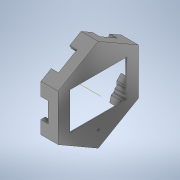
# Autodesk Inventor part: Hexagone
Saved by Autodesk Inventor 2020 (Build 240168000, 168)
## iProperties
Created: 2020-04-08
Part Number: Hexagone
Material: Silicon Nitride
Document SubType Name: Modeling
Designer: Samuele
Density: 3.18 g/cm^3
Appearance: Chrome - Polished Black
Author: Samuele
## iProperties of the stored document _3DPrint.ipt
Created: 2020-04-30
Part Number: _3DPrint
Material: Generic
Document SubType Name: Modeling
Designer: Samuele
Density: 1 g/cm^3
Appearance: Default
Author: Samuele
Autodesk Inventor part; units mm, degrees
ref_plane "YZ Plane" through (0, 0, 0) normal (1, 0, 0) x (0, 1, 0)
ref_plane "XZ Plane" through (0, 0, 0) normal (0, 1, 0) x (-1, 0, 0)
ref_plane "XY Plane" through (0, 0, 0) normal (0, 0, 1) x (1, 0, 0)
sketch "Sketch6" plane through (0, 0, 0) normal (0, 1, 0) x (-1, 0, 0)
  line L0 (4.5, -5.6) -> (60.5, -5.6)
  line L1 (60.5, -5.6) -> (60.5, -91.4)
  line L2 (4.5, -91.4) -> (4.5, -5.6)
  line L3 (65.1201, -97) -> (0, -97)
  line L4 (0, -97) -> (0, 0)
  line L5 (0, 0) -> (65.1201, 0)
  line L6 (65.1201, 0) -> (65.1201, -97)
  line L7 (60.5, -91.4) -> (4.5, -91.4)
  line L8 (102.5, -48.5) -> (-37.5, -48.5)
  line L9 (32.5, -118.5) -> (32.5, 21.5)
  circle A0 centre (32.5, -48.5) radius 70
  line L10 (102.5, -48.5) -> (67.5, -109.1218)
  line L11 (67.5, -109.1218) -> (-2.5, -109.1218)
  line L12 (-2.5, -109.1218) -> (-37.5, -48.5)
  line L13 (-37.5, -48.5) -> (-2.5, 12.1218)
  line L14 (-2.5, 12.1218) -> (67.5, 12.1218)
  line L15 (67.5, 12.1218) -> (102.5, -48.5)
  line L16 (32.5, 12.1218) -> (85, -18.1891)
  line L17 (85, -18.1891) -> (85, -78.8109)
  line L18 (85, -78.8109) -> (32.5, -109.1218)
  line L19 (32.5, -109.1218) -> (-20, -78.8109)
  line L20 (-20, -78.8109) -> (-20, -18.1891)
  line L21 (-20, -18.1891) -> (32.5, 12.1218)
  line L22 (32.5, 12.1218) -> (47.5, 12.1218)
  line L23 (47.5, 12.1218) -> (47.5, 5.6218)
  line L24 (47.5, 5.6218) -> (17.5, 5.6218)
  line L25 (17.5, 5.6218) -> (17.5, 12.1218)
  line L26 (47.5, 5.6218) -> (56.6924, 5.6218) construction
  line L27 (17.5, 8.8718) -> (19.5, 8.8718)
  line L28 (47.5, 8.8718) -> (45.5, 8.8718)
  line L29 (45.5, 8.8718) -> (45.5, 10.1218)
  line L30 (45.5, 10.1218) -> (19.5, 10.1218)
  line L31 (19.5, 10.1218) -> (19.5, 7.6218)
  line L32 (19.5, 7.6218) -> (45.5, 7.6218)
  line L33 (45.5, 7.6218) -> (45.5, 10.1218)
  line L34 (67.5, 12.1218) -> (32.5, -48.5)
  line L35 (32.5, -48.5) -> (67.5, -109.1218)
  line L36 (47.5, 5.6218) -> (56.6924, 5.6218)
  line L37 (17.5, 5.6218) -> (11, 5.6218)
  line L38 (17.5, 12.1218) -> (11, 5.6218)
  line L39 (17.5, 12.1218) -> (26.6924, 12.1218) construction
  line L40 (47.5, 12.1218) -> (54, 5.6218)
  line L41 (85, -18.1891) -> (77.5, -5.1987)
  line L42 (77.5, -5.1987) -> (71.8708, -8.4487)
  line L43 (71.8708, -8.4487) -> (86.8708, -34.4295)
  line L44 (86.8708, -34.4295) -> (92.5, -31.1795)
  line L45 (71.8708, -8.4487) -> (67.2746, -0.4879) construction
  line L46 (89.6854, -32.8045) -> (88.6854, -31.0724)
  line L47 (74.6854, -6.8237) -> (75.6854, -8.5558)
  line L48 (75.6854, -8.5558) -> (76.7679, -7.9308)
  line L49 (76.7679, -7.9308) -> (89.7679, -30.4474)
  line L50 (89.7679, -30.4474) -> (87.6029, -31.6974)
  line L51 (87.6029, -31.6974) -> (74.6029, -9.1808)
  line L52 (74.6029, -9.1808) -> (76.7679, -7.9308)
  line L53 (71.8708, -8.4487) -> (67.2746, -0.4879)
  line L54 (86.8708, -34.4295) -> (90.1208, -40.0587)
  line L55 (92.5, -31.1795) -> (90.1208, -40.0587)
  line L56 (92.5, -31.1795) -> (87.9038, -23.2187) construction
  line L57 (77.5, -5.1987) -> (68.6208, -2.8196)
  line L58 (71.8708, -88.5513) -> (67.2746, -96.5121) construction
  line L59 (74.6854, -90.1763) -> (75.6854, -88.4442)
  line L60 (74.6029, -87.8192) -> (76.7679, -89.0692)
  line L61 (77.5, -91.8013) -> (71.8708, -88.5513)
  line L62 (77.5, -91.8013) -> (68.6208, -94.1804)
  line L63 (71.8708, -88.5513) -> (67.2746, -96.5121)
  line L64 (76.7679, -89.0692) -> (89.7679, -66.5526)
  line L65 (87.6029, -65.3026) -> (74.6029, -87.8192)
  line L66 (71.8708, -88.5513) -> (86.8708, -62.5705)
  line L67 (89.7679, -66.5526) -> (87.6029, -65.3026)
  line L68 (89.6854, -64.1955) -> (88.6854, -65.9276)
  line L69 (86.8708, -62.5705) -> (92.5, -65.8205)
  line L70 (86.8708, -62.5705) -> (90.1208, -56.9413)
  line L71 (92.5, -65.8205) -> (90.1208, -56.9413)
  line L72 (94.9944, -48.5) -> (63.7472, -102.6218)
  line L73 (63.7472, -102.6218) -> (1.2528, -102.6218)
  line L74 (1.2528, -102.6218) -> (-29.9944, -48.5)
  line L75 (-29.9944, -48.5) -> (1.2528, 5.6218)
  line L76 (1.2528, 5.6218) -> (63.7472, 5.6218)
  line L77 (63.7472, 5.6218) -> (94.9944, -48.5)
  line L78 (74.6029, -87.8192) -> (72.8708, -86.8192)
  line L79 (87.6029, -65.3026) -> (85.8708, -64.3026)
  line L80 (87.6029, -31.6974) -> (85.8708, -32.6974)
  line L81 (74.6029, -9.1808) -> (72.8708, -10.1808)
  line L82 (45.5, 7.6218) -> (45.5, 5.6218)
  line L83 (19.5, 7.6218) -> (19.5, 5.6218)
  line L84 (60.5, -91.4) -> (4.4985, -91.4)
  line L85 (4.4985, -97) -> (60.5, -97)
  line L86 (60.5, -5.6) -> (4.4985, -5.6)
  line L87 (4.4985, 0) -> (60.5, 0)
  line L88 (-29.9944, -48.5) -> (-22.9944, -48.5)
  line L89 (-29.9944, -48.5) -> (-28.2944, -48.5)
  line L90 (-28.2944, -48.5) -> (-22.9944, -48.5)
  circle A1 centre (-26.9944, -48.5) radius 1.5
  line L91 (-29.9944, -48.5) -> (-23.9944, -48.5)
  line L92 (-23.9944, -48.5) -> (-26.9944, -53.6962)
  line L93 (-23.9944, -48.5) -> (-26.9944, -43.3038)
  line L94 (32.4993, -5.6) -> (32.4993, 0)
  line L95 (32.4993, -91.4) -> (32.4993, -97)
  line L96 (60.5, -5.6) -> (60.5, 0)
  line L97 (4.4985, -5.6) -> (4.4985, 0)
  line L98 (4.4985, -91.4) -> (4.4985, -97)
  line L99 (60.5, -91.4) -> (60.5015, -97)
  point P0 (19.5, 8.8718)
  point P1 (88.6854, -31.0724)
  point P2 (88.6854, -65.9276)
  point P3 (75.6854, -8.5558)
  point P4 (19.5, 5.6218)
  point P5 (45.5, 5.6218)
  point P6 (85.8708, -32.6974)
  point P7 (72.8708, -10.1808)
  point P8 (72.8708, -86.8192)
  point P9 (85.8708, -64.3026)
  point P10 (4.5, -91.4)
  point P11 (4.5, -5.6)
  point P12 (-27.5473, -52.7386)
  point P13 (-28.2775, -45.5261)
  dimension "d44" = 97
  dimension "d77" = 140
  dimension "d87" = 15
  dimension "d88" = 6.5
  dimension "d89" = 30
  dimension "d91" = 2
  dimension "d92" = 2
  dimension "d95" = 1.25
  dimension "d96" = 26
  dimension "d97" = 2.5
  dimension "d98" = 26
  dimension "d99" = 135
  dimension "d100" = 0
  dimension "d114" = 1.7
  dimension "d117" = 3
  dimension "d121" = 3
  dimension "d123" = 6
  dimension "d124" = 85.8
  constraints: 200 end point, 37 symmetric about line, 23 point on line, 11 horizontal, 11 perpendicular, 9 midpoint, 7 parallel, 5 vertical, 4 collinear, 4 point on circle, 3 coincident, 2 centre point, 2 equal length, 1 horizontal alignment, 41 other
  measures "d44" distance of L5.end L3.start
  measures "d77" diameter of A0
  measures "d87" distance of L16.start L22.end
  measures "d88" distance of L22.end L23.end
  measures "d89" distance of L23.end L24.end
  measures "d91" distance of L27.start L27.end
  measures "d92" distance of L28.start L28.end
  measures "d95" distance of L28.end L29.end
  measures "d96" distance of L29.end L30.end
  measures "d97" distance of L30.end L31.end
  measures "d98" distance of L31.end L32.end
  measures "d99" angle of L38 L39
  measures "d100" distance of L25.end L38.start
  measures "d114" distance of L74.end L89.end
  measures "d117" diameter of A1
  measures "d121" distance of L74.end A1.centre
  measures "d123" distance of L74.end L91.end
  measures "d124" distance between parallel lines of L7 L0
extrude "Fronte" add sketch "Sketch6" along normal blind 1 contours L97 L21 L5 L9 L0 | L2 L8 L4 L21 L97 | L9 L5 L16 L34 L0 | L2 L98 L19 L4 L8 | L97 L5 L21 | L21 L4 L5 L97 | L34 L16 L96 L0 | L9 L24 L16 L5 | L5 L21 L24 L9 | L7 L9 L3 L19 L98 | L8 L20 L75 L21 L4 | L4 L19 L74 L20 L8 | L21 L75 L76 L37 L24 L5 L4 | L96 L16 L6 L8 L1 | L34 L96 L16 | L16 L5 L34 | L8 L6 L18 L99 L1 | L7 L35 L18 L3 L9 | L7 L99 L18 L35 | L16 L24 L36 L76 L34 L5 | L24 L21 L32 L9 | L9 L32 L16 L24 | L98 L3 L4 L19 | L19 L3 L98 | L4 L3 L19 L73 L74 | L20 L74 L92 L8 | L8 L93 L75 L20 | L75 L20 L21 | L21 L13 L14 L38 L76 L75 | L24 L83 L32 L21 | L96 L5 L6 L16 | L34 L77 L53 L43 L16 L6 L5 | L8 L17 L66 L18 L6 | L6 L16 L43 L17 L8 | L9 L73 L19 L3 | L3 L18 L73 L9 | L35 L3 L18 | L18 L99 L35 | L16 L32 L82 L24 | L32 L21 L30 L9 | L9 L30 L16 L32 | L74 L73 L19 L11 L12 | L19 L20 L74 | L20 L12 L8 L74 | L75 L8 L13 L20 | L32 L31 L30 L21 | L24 L25 L27 L31 L83 | L76 L36 L40 L14 L34 | L34 L15 L57 L53 L77 | L18 L6 L3 L99 | L18 L66 L63 L72 L35 L3 L6 | L17 L43 L54 L77 L8 | L8 L72 L70 L66 L17 | L3 L35 L73 L18 | L73 L18 L9 | L9 L19 L73 | L16 L30 L29 L33 L32 | L82 L33 L28 L23 L24 | L30 L21 L9 | L9 L16 L30 | L92 L74 L8 A1 | L8 A1 L75 L93 | L38 L25 L37 | L30 L31 L27 L25 L14 L21 | L43 L81 L51 L16 | L16 L51 L17 L43 | L66 L17 L65 L18 | L18 L65 L78 L66 | L77 L55 L15 L8 | L8 L10 L71 L72 | L17 L51 L80 L43 | L66 L79 L65 L17 | L73 L35 L11 L18 | L72 L63 L62 L10 L35 | L16 L14 L23 L28 L29 L30 | L23 L40 L36 | A1 L8 | L8 A1 | L51 L52 L48 L49 L16 | L16 L49 L17 L51 | L43 L42 L47 L52 L81 | L15 L16 L49 L48 L47 L42 | L42 L53 L57 | L65 L17 L64 L18 | L18 L64 L60 L65 | L78 L60 L59 L61 L66 | L71 L69 L70 | L54 L44 L55 | L17 L49 L50 L51 | L80 L50 L46 L44 L43 | L65 L67 L64 L17 | L66 L69 L68 L67 L79 | L16 L17 L49 | L10 L17 L64 L67 L68 L69 | L44 L46 L50 L49 L17 L15 | L64 L17 L18 | L18 L10 L61 L59 L60 L64 | L61 L62 L63
extrude "Esterno" add sketch "Sketch6" against normal blind 25 contours L75 L20 L21 | L21 L13 L14 L38 L76 L75 | L74 L73 L19 L11 L12 | L19 L20 L74 | L20 L12 L8 L74 | L75 L8 L13 L20 | L76 L36 L40 L14 L34 | L34 L15 L57 L53 L77 | L73 L18 L9 | L9 L19 L73 | L77 L55 L15 L8 | L8 L10 L71 L72 | L73 L35 L11 L18 | L72 L63 L62 L10 L35
extrude "Strip" add sketch "Sketch6" against normal blind 10 contours L24 L21 L32 L9 | L9 L32 L16 L24 | L24 L83 L32 L21 | L16 L32 L82 L24 | L24 L25 L27 L31 L83 | L82 L33 L28 L23 L24 | L30 L21 L9 | L9 L16 L30 | L38 L25 L37 | L30 L31 L27 L25 L14 L21 | L43 L81 L51 L16 | L16 L51 L17 L43 | L66 L17 L65 L18 | L18 L65 L78 L66 | L17 L51 L80 L43 | L66 L79 L65 L17 | L16 L14 L23 L28 L29 L30 | L23 L40 L36 | L43 L42 L47 L52 L81 | L15 L16 L49 L48 L47 L42 | L42 L53 L57 | L78 L60 L59 L61 L66 | L71 L69 L70 | L54 L44 L55 | L80 L50 L46 L44 L43 | L66 L69 L68 L67 L79 | L16 L17 L49 | L10 L17 L64 L67 L68 L69 | L44 L46 L50 L49 L17 L15 | L64 L17 L18 | L18 L10 L61 L59 L60 L64 | L61 L62 L63
sketch "Sketch7" plane through (0, -25, 0) normal (0, -1, 0) x (1, 0, 0)
  line L0 (-17.5, 12.1218) -> (-17.5, -109.1218)
  line L1 (-67.5, -109.1218) -> (2.5, -109.1218) projected
  line L2 (-47.5, 12.1218) -> (-67.5, 12.1218) projected
  line L3 (-47.5, 12.1218) -> (-47.5, -109.1218)
  line L4 (-77.5, -91.8013) -> (-67.5, -109.1218) projected
  line L5 (-77.5, -91.8013) -> (27.5, -31.1795)
  line L6 (2.5, 12.1218) -> (37.5, -48.5) projected
  line L7 (-92.5, -65.8205) -> (-90.1208, -56.9413) projected
  line L8 (-92.5, -65.8205) -> (12.5, -5.1987)
  line L9 (-77.5, -5.1987) -> (27.5, -65.8205)
  line L10 (37.5, -48.5) -> (2.5, -109.1218) projected
  line L11 (-92.5, -31.1795) -> (11.423, -93.6666)
  line L12 (27.5, -31.1795) -> (12.5, -5.1987)
  line L13 (27.5, -65.8205) -> (11.423, -93.6666)
  line L14 (-1.2528, -102.6218) -> (29.9944, -48.5) projected
  line L15 (5.8516, -90.3166) -> (21.8708, -62.5705)
  line L16 (-47.5, -109.1218) -> (-17.5, -109.1218)
  line L17 (-17.5, -109.1218) -> (-17.5, -102.6218)
  line L18 (-17.5, -102.6218) -> (-47.5, -102.6218)
  line L19 (-47.5, -102.6218) -> (-47.5, -109.1218)
  line L20 (5.5339, -9.2206) -> (17.5, -36.953)
  point P0 (0, 0)
  point P1 (6.9325, -8.4131)
  point P2 (21.9325, -34.3939)
  constraints: 28 end point, 13 point on line, 3 parallel, 2 vertical, 1 horizontal, 1 perpendicular
extrude "Passacavi" cut sketch "Sketch7" against normal blind 11 contours L0 L1 L3 L18 | L14 L9 L10 L11 | L20 L8 L6 L5
extrude "ScavoStrip" cut sketch "Sketch6" against normal blind 5 contours L24 L21 L32 L9 | L9 L32 L16 L24 | L24 L83 L32 L21 | L16 L32 L82 L24 | L43 L81 L51 L16 | L16 L51 L17 L43 | L66 L17 L65 L18 | L18 L65 L78 L66 | L17 L51 L80 L43 | L66 L79 L65 L17
extrude "ScreenDist0.8" add sketch "Sketch6" against normal blind 0.8 contours L97 L21 L5 L9 L0 | L9 L5 L16 L34 L0 | L97 L5 L21 | L34 L16 L96 L0 | L34 L96 L16 | L16 L5 L34
extrude "SupportoViti" add sketch "Sketch6" against normal blind 23 contours L92 L74 L8 A1 | L8 A1 L75 L93
pattern_circular "RipetizioneSupports" count 6 over 360 about axis through (-32.5, 0, -48.5) along (0, -1, 0) of "SupportoViti"
chamfer "Smusso interno" distance 1 angle 45 30 edges at (14.3708, 0, -21.4391) (-1.2528, 0, 0.4256) (-5.7528, 0, 3.0237) (-13.3764, 0, 5.6218) (-19.5, 0, 7.8718) (-32.5, 0, 10.1218) (-45.5, 0, 7.8718) (-51.6236, 0, 5.6218) (-59.2472, 0, 3.0237) (-63.7472, 0, 0.4256) (-69.809, 0, -4.8776) (-74.8194, 0, -9.0558) (25.4944, 0, -45.9019) (25.4944, 0, -51.0981) (-83.2679, 0, -19.1891) (-87.8194, 0, -31.5724) (-88.9326, 0, -38.0006) (-90.4944, 0, -45.9019) (-90.4944, 0, -51.0981) (-88.9326, 0, -58.9994) (-87.8194, 0, -65.4276) (-83.2679, 0, -77.8109) (14.3708, 0, -75.5609) (-1.2528, 0, -97.4256) (-5.7528, 0, -100.0237) (-32.5, 0, -102.6218) (-59.2472, 0, -100.0237) (-63.7472, 0, -97.4256) (-69.809, 0, -92.1224) (-74.8194, 0, -87.9442)
fillet "RaccordoSupports" radius 1 18 edges at (1.7472, -12, 0.4256) (-7.2528, -12, 5.6218) (26.9944, -12, -43.3038) (23.9944, -12, -48.5) (26.9944, -12, -53.6962) (-4.2528, -12, 0.4256) (-57.7472, -12, 5.6218) (-60.7472, -12, 0.4256) (-66.7472, -12, 0.4256) (-91.9944, -12, -53.6962) (-88.9944, -12, -48.5) (-91.9944, -12, -43.3038) (-57.7472, -12, -102.6218) (-60.7472, -12, -97.4256) (-66.7472, -12, -97.4256) (1.7472, -12, -97.4256) (-4.2528, -12, -97.4256) (-7.2528, -12, -102.6218)
sketch "Sketch9" plane through (0, 1, 0) normal (0, 1, 0) x (1, 0, 0)
  line L0 (-67.5, 109.1218) -> (-102.5, 48.5) projected
  line L1 (-102.5, 48.5) -> (-60.5, 48.5)
  line L2 (-60.5, 5.6) -> (-60.5, 91.4) projected
  line L3 (-78.5, 38.5) -> (-78.5, 58.5)
  point P0 (0, 0)
  point P1 (-78.5, 48.5)
  point P2 (-81.5, 48.5)
  point P3 (-78.5, 48.5)
  dimension "d132" = 20
  dimension "d133" = 18
  constraints: 4 end point, 3 midpoint, 1 coincident, 1 horizontal alignment, 1 vertical
  measures "d132" distance of L3.start L3.end
  measures "d133" distance between parallel lines of L2 L3
hole "ForoPulsante" at (-78.5, 1, -48.5) direction (0, -1, 0) diameter 3 end through all
body "Solid3"
